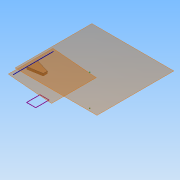
# Autodesk Inventor part: 40523209
Saved by Autodesk Inventor 2015 (Build 190159000, 159)
## iProperties
Created: 2018-05-07
Part Number: 40523209
Material: 一般
Document SubType Name: Modeling
Designer: 王博聖
Density: 1 g/cm^3
Appearance: 預設
Author: 王博聖
Autodesk Inventor part; units mm, degrees
ref_plane "YZ Plane" through (0, 0, 0) normal (1, 0, 0) x (0, 1, 0)
ref_plane "XZ Plane" through (0, 0, 0) normal (0, 1, 0) x (-1, 0, 0)
ref_plane "XY Plane" through (0, 0, 0) normal (0, 0, 1) x (1, 0, 0)
sketch "草圖1" plane through (0, 0, 0) normal (0, 0, 1) x (1, 0, 0)
  line L0 (-59.6872, -28.0111) -> (-79.2339, -28.0111)
  line L1 (-79.2339, -28.0111) -> (-79.2339, -56.633)
  line L2 (-79.2339, -56.633) -> (-59.6872, -56.633)
  line L3 (-59.6872, -56.633) -> (-59.6872, -28.0111)
  point P0 (0, 0)
  constraints: 8 end point, 2 parallel, 1 horizontal, 1 perpendicular
ref_plane "工作平面1" through (0, 0, 67.25) normal (0, 0, 1) x (1, 0, 0)
sketch "草圖2" plane through (0, 0, 67.25) normal (0, 0, 1) x (1, 0, 0)
  line L0 (-78, -31.4361) -> (-78, 5.7991) projected
  line L1 (-78, 5.7991) -> (-78, -80.9826)
  point P0 (0, 0)
  constraints: 2 end point, 1 vertical
ref_plane "工作平面2" through (-78, 5.7991, 67.25) normal (0.0871557, 0, 0.9961947) x (0, -1, 0)
sketch "草圖3" plane through (-78, 5.7991, 67.25) normal (0.0871557, 0, 0.9961947) x (0, -1, 0)
  line L0 (62.4321, 4.6321) -> (62.4321, 24.1044) projected
  line L1 (34.5073, 0.4668) -> (56.728, 0.4668)
  line L2 (56.728, 0.4668) -> (49.3043, 28.2093)
  line L3 (34.5073, 0.4668) -> (40.6164, 28.2093)
  line L4 (40.6164, 28.2093) -> (49.3043, 28.2093)
  point P0 (5.7991, 83.5644)
  point P1 (33.8102, 24.1044)
  constraints: 8 end point, 2 horizontal
extrude "擠出1" add sketch "草圖3" against normal blind 5
